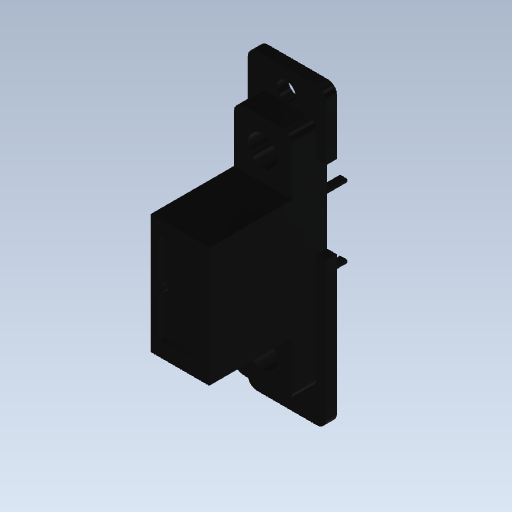
# Autodesk Inventor part: Line Tracker PCB
Saved by Autodesk Inventor 2020 (Build 240168000, 168)
## iProperties
Created: 2012-03-30
Part Number: Line Tracker PCB
Document SubType Name: Modeling
Designer: Autodesk Inc.
Density: 1 g/cm^3
Catalog Web Link: http://www.vexrobotics.com/276-2154.html
Vendor: VEX
Material: 一般
Appearance: 有光泽 - 黑色
Category: Sensors
Company: Autodesk Inc.
Author: Autodesk Inc.
Autodesk Inventor part; units mm, degrees
ref_plane "YZ Plane" through (0, 0, 0) normal (1, 0, 0) x (0, 1, 0)
ref_plane "XZ Plane" through (0, 0, 0) normal (0, 1, 0) x (-1, 0, 0)
ref_plane "Work Plane4" through (0, 0, -0.1524) normal (0, 0, 1) x (1, 0, 0)
sketch "Sketch4" plane through (0, 0, -0.1524) normal (0, 0, 1) x (1, 0, 0)
  line L0 (3.3587, -7.5194) -> (-3.2453, -7.5194) projected
  line L1 (-3.2453, -7.5194) -> (-3.2453, 5.8918) projected
  line L2 (-3.2453, 5.8918) -> (3.3587, 5.8918) projected
  line L3 (3.3587, 5.8918) -> (3.3587, -7.5194) projected
  line L4 (-4.3472, -17.7639) -> (-4.3472, 17.7639) projected
  line L5 (4.3472, -17.7639) -> (-4.3472, -17.7639) projected
  line L6 (4.3472, 17.7639) -> (4.3472, -17.7639) projected
  line L7 (-4.3472, 17.7639) -> (4.3472, 17.7639) projected
  line L8 (-3.1183, 5.6886) -> (3.2317, 5.6886)
  line L9 (3.2317, 5.6886) -> (3.2317, -7.3162)
  line L10 (3.2317, -7.3162) -> (-3.1183, -7.3162)
  line L11 (-3.1183, -7.3162) -> (-3.1183, 5.6886)
  point P0 (0, 0)
  point P1 (3.2317, -0.8138)
  point P2 (3.3587, -0.8138)
  point P3 (0.0567, 5.6886)
  point P4 (0.0567, 5.8918)
  dimension "d15" = 13.0048
  dimension "d16" = 6.35
  constraints: 8 end point, 4 midpoint, 2 parallel, 1 horizontal, 1 horizontal alignment, 1 perpendicular, 1 vertical alignment
  measures "d15" distance of L8.end L9.end
  measures "d16" distance of L8.start L8.end
extrude "Extrusion3" add sketch "Sketch4" against normal blind 9.0424 contours L8 L9 L10 L11
sketch "Sketch5" plane through (0, 0, -9.1948) normal (0, 0, -1) x (-1, 0, 0)
  line L0 (3.1183, 11.8608) -> (-3.2317, 11.8608)
  line L1 (-3.2317, 11.8608) -> (-3.2317, -13.4884)
  line L2 (-3.2317, -13.4884) -> (3.1183, -13.4884)
  line L3 (3.1183, -13.4884) -> (3.1183, 11.8608)
  line L4 (-3.2317, 5.6886) -> (-3.2317, -7.3162) projected
  line L5 (3.1183, 5.6886) -> (-3.2317, 5.6886) projected
  point P0 (0, 0)
  point P1 (-3.2317, -0.8138)
  point P2 (-3.2317, -0.8138)
  point P3 (-0.0567, 5.6886)
  point P4 (-0.0567, 11.8608)
  dimension "d19" = 25.3492
  constraints: 8 end point, 4 midpoint, 2 parallel, 1 coincident, 1 collinear, 1 horizontal, 1 perpendicular, 1 vertical alignment
  measures "d19" distance of L0.end L1.end
extrude "Extrusion4" add sketch "Sketch5" along normal blind 2.5908
fillet "Fillet2" radius 0.9906 4 edges at (-3.1183, 11.8608, -10.4902) (3.2317, 11.8608, -10.4902) (3.2317, -13.4884, -10.4902) (-3.1183, -13.4884, -10.4902)
sketch "Sketch6" plane through (0, 0, -11.7856) normal (0, 0, -1) x (-1, 0, 0)
  arc A0 (2.1277, -13.4884) -> (3.1183, -12.4978) centre (2.1277, -12.4978) ccw projected
  line L0 (3.1183, 10.8702) -> (3.1183, -12.4978) projected
  arc A1 (3.1183, 10.8702) -> (2.1277, 11.8608) centre (2.1277, 10.8702) ccw projected
  arc A2 (-2.2411, 11.8608) -> (-3.2317, 10.8702) centre (-2.2411, 10.8702) ccw projected
  line L1 (-3.2317, -12.4978) -> (-3.2317, 10.8702) projected
  arc A3 (-3.2317, -12.4978) -> (-2.2411, -13.4884) centre (-2.2411, -12.4978) ccw projected
  line L2 (2.1277, -13.4884) -> (-2.2411, -13.4884) projected
  line L3 (4.1978, 15.1882) -> (-4.3112, 15.1882)
  line L4 (-4.3112, 15.1882) -> (-4.3112, -16.8158)
  line L5 (-4.3112, -16.8158) -> (4.1978, -16.8158)
  line L6 (4.1978, -16.8158) -> (4.1978, 15.1882)
  line L7 (-3.2317, 5.6886) -> (-3.2317, -7.3162) projected
  line L8 (2.1277, 11.8608) -> (-2.2411, 11.8608) projected
  point P0 (0, 0)
  point P1 (-3.2317, -0.8138)
  point P2 (-4.3112, -0.8138)
  point P3 (-0.0567, 11.8608)
  point P4 (-0.0567, 15.1882)
  dimension "d24" = 32.004
  dimension "d25" = 8.509
  constraints: 8 end point, 4 midpoint, 2 parallel, 1 horizontal, 1 horizontal alignment, 1 perpendicular, 1 vertical alignment
  measures "d24" distance of L3.end L4.end
  measures "d25" distance of L3.start L3.end
extrude "Extrusion5" add sketch "Sketch6" along normal blind 1.1938 contours L2 A3 L1 A2 L8 A1 L0 A0 | L6 L5 L4 L3
fillet "Fillet3" radius 0.9906 4 edges at (-4.1978, 15.1882, -12.3825) (4.3112, 15.1882, -12.3825) (-4.1978, -16.8158, -12.3825) (4.3112, -16.8158, -12.3825)
sketch "Sketch7" plane through (0, 0, -12.9794) normal (0, 0, -1) x (-1, 0, 0)
  circle A0 centre (-0.0045, 8.6858) radius 1.9939 projected
  circle A1 centre (-0.0045, -10.3134) radius 1.9939 projected
  point P0 (0, 0)
hole "Hole2" at (0.0045, 8.6858, -12.9794) at (0.0045, -10.3134, -12.9794) direction (0, 0, 1) diameter 3.2004 depth 3.7846
sketch "Sketch8" plane through (0, 0, -12.9794) normal (0, 0, -1) x (-1, 0, 0)
  circle A0 centre (-0.0045, -10.3134) radius 1.6002 projected
  circle A1 centre (-0.0045, 8.6858) radius 1.6002 projected
  line L0 (-4.3112, -15.8252) -> (-4.3112, 14.1976) projected
  line L1 (-0.0045, -14.6187) -> (-0.0045, 12.9911) construction
  point P0 (0, 0)
  point P1 (-0.0045, -0.8138)
  point P2 (-4.3112, -0.8138)
  dimension "d36" = 27.6098
  constraints: 2 end point, 2 midpoint, 2 vertical alignment, 1 horizontal alignment, 1 parallel
  measures "d36" distance of L1.end L1.start
hole "Hole3" at (0.0045, -14.6187, -12.9794) at (0.0045, 12.9911, -12.9794) direction (0, 0, 1) diameter 2.0066 end up to surface
sketch "Sketch9" plane through (0, 0, -12.9794) normal (0, 0, -1) x (-1, 0, 0)
  line L0 (3.2072, -16.8158) -> (-3.3206, -16.8158) projected
  line L1 (-4.3112, -15.8252) -> (-4.3112, 14.1976) projected
  line L2 (-0.933, -4.7762) -> (-1.7204, -4.7762)
  line L3 (-1.7204, -4.7762) -> (-1.7204, -4.4714)
  line L4 (-1.7204, -4.4714) -> (-0.933, -4.4714)
  line L5 (-0.933, -4.4714) -> (-0.933, -4.7762)
  point P0 (0, 0)
  dimension "d44" = 0.7874
  dimension "d45" = 0.3048
  dimension "d46" = 12.0396
  dimension "d47" = 2.5908
  constraints: 8 end point, 2 parallel, 1 horizontal, 1 perpendicular
  measures "d44" distance of L3.end L4.end
  measures "d45" distance of L2.end L3.end
  measures "d46" distance between parallel lines of L2 L0
  measures "d47" distance between parallel lines of L1 L3
extrude "Extrusion6" add sketch "Sketch9" along normal blind 3.7084
pattern_linear "Rectangular Pattern1" count 2 spacing 7.62 along (0, 1, 0) count 2 spacing 2.54 along (-1, 0, 0) of "Extrusion6"
sketch "Sketch10" plane through (0, 0, -12.9794) normal (0, 0, -1) x (-1, 0, 0)
  line L0 (-3.3206, 15.1882) -> (3.2072, 15.1882) projected
  line L1 (-4.3112, -15.8252) -> (-4.3112, 14.1976) projected
  line L2 (-3.219, -0.8138) -> (-4.3112, -0.8138)
  line L3 (-4.3112, -0.8138) -> (-4.3112, 8.1778)
  line L4 (-4.3112, 8.1778) -> (-3.219, 8.1778)
  line L5 (-3.219, 8.1778) -> (-3.219, -0.8138)
  point P0 (0, 0)
  dimension "d56" = 7.0104
  dimension "d57" = 8.9916
  dimension "d58" = 1.0922
  constraints: 8 end point, 2 parallel, 1 collinear, 1 horizontal, 1 perpendicular
  measures "d56" distance between parallel lines of L4 L0
  measures "d57" distance of L2.end L3.end
  measures "d58" distance of L3.end L4.end
extrude "Extrusion7" cut sketch "Sketch10" against normal up to surface (1.1938 mm away)
sketch "Sketch11" plane through (0, 0, -0.1524) normal (0, 0, 1) x (1, 0, 0)
  line L0 (-3.1183, 5.6886) -> (3.2317, 5.6886) projected
  line L1 (3.2317, -7.3162) -> (-3.1183, -7.3162) projected
  line L2 (-3.1133, 5.6862) -> (3.2267, 5.6862)
  line L3 (-3.1133, -7.3138) -> (-3.1133, 5.6862)
  line L4 (-3.1133, -7.3138) -> (3.2267, -7.3138)
  line L5 (3.2267, 5.6862) -> (3.2267, -7.3138)
  arc A0 (2.3267, -0.3138) -> (2.3267, -1.3138) centre (2.3267, -0.8138) ccw
  line L6 (2.3267, -1.3138) -> (2.3267, -5.7138)
  line L7 (2.3267, -5.7138) -> (-2.2133, -5.7138)
  line L8 (-2.2133, -5.7138) -> (-2.2133, -1.3138)
  arc A1 (-2.2133, -1.3138) -> (-2.2133, -0.3138) centre (-2.2133, -0.8138) ccw
  line L9 (-2.2133, -0.3138) -> (-2.2133, 4.0862)
  line L10 (-2.2133, 4.0862) -> (2.3267, 4.0862)
  line L11 (2.3267, 4.0862) -> (2.3267, -0.3138)
  line L12 (0.0567, -7.3162) -> (0.0567, 5.6886) construction
  point P0 (0, 0)
  point P1 (0.0567, -0.8138)
  point P2 (0.0567, -0.8138)
  constraints: 22 end point, 4 point on circle, 3 midpoint, 2 centre point
extrude "Extrusion8" cut sketch "Sketch11" against normal blind 0.508 contours A0 L6 L7 L8 A1 L9 L10 L11
body "Solid2"
